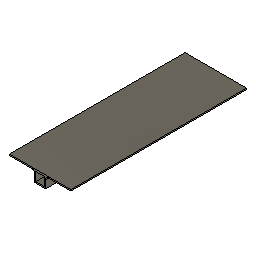
electronic_component_holder better (Autodesk Fusion 360 design; units mm, degrees)
Autodesk Fusion 360 part; units mm, degrees
sketch "Sketch1" plane through (0, 0, 0) normal (0, 0, 1) x (1, 0, 0)
  line L0 (0, 0) -> (17, 0)
  line L1 (17, 0) -> (17, 200)
  line L2 (17, 200) -> (0, 200)
  line L3 (0, 200) -> (0, 0)
  line L4 (5, 0) -> (5, 200)
  line L5 (12, 0) -> (12, 200)
  dimension "d1" = 17
  dimension "d2" = 200
  dimension "d3" = 200
  dimension "d4" = 7
  dimension "d5" = 200
  constraint horizontal L0
  constraint vertical L1
  constraint horizontal L2
  constraint vertical L3
  constraint coincident L0.start L3.end
  constraint coincident L0 L4.start
  constraint perpendicular L0 L5
  measures "d1" distance of L0.start L0.end
  measures "d2" distance of L0.start L2.end
  measures "d3" distance of L4.start L4.end
  measures "d4" distance of L4.start L5.start
  measures "d5" distance of L5.start L5.end
extrude "Extrude1" add sketch "Sketch1" along normal blind 5
sketch "Sketch2" plane through (0, 0, 5) normal (0, 0, 1) x (-1, 0, 0)
  line L0 (0, -200) -> (0, 0)
  line L1 (0, 0) -> (-17, 0)
  line L2 (-17, 0) -> (-17, -200)
  line L3 (-17, -200) -> (0, -200)
  line L4 (-5, 0) -> (-5, -200)
  line L5 (-12, 0) -> (-12, -200)
  dimension "d8" = 5
  dimension "d9" = 7
  dimension "d10" = 200
  dimension "d11" = 200
  constraint perpendicular L1 L4
  constraint perpendicular L1 L5
  measures "d8" distance of L0.end L4.start
  measures "d9" distance of L4.start L5.start
  measures "d10" distance of L4.start L4.end
  measures "d11" distance of L5.start L5.end
extrude "Extrude2" add sketch "Sketch2" along normal blind 12 contours L0 L1 L3 L4 | L1 L2 L3 L5
sketch "Sketch3" plane through (12, 0, 0) normal (-1, 0, 0) x (0, -1, 0)
  line L0 (-200, 5) -> (0, 5)
  line L1 (0, 5) -> (0, 17)
  line L2 (0, 17) -> (-200, 17)
  line L3 (-200, 17) -> (-200, 5)
  line L4 (0, 17) -> (0, 12)
  line L5 (0, 12) -> (-200, 12)
  dimension "d14" = 200
  constraint coincident L1.end L2.start
  constraint coincident L1 L4.end
  constraint perpendicular L2 L4
  constraint perpendicular L4 L5
  measures "d14" distance of L4.end L5.end
extrude "Extrude3" add sketch "Sketch3" along normal blind 7 contours L1 L2 L3 L4 L5
move_face "OffsetFaces1" offset -0.5 4 faces at (12, 133.3333, 9.6667) (9.6667, 66.6667, 12) (5, 133.3333, 9.6667) (7.3333, 133.3333, 5)
sketch "Sketch4" plane through (0, 0, 17) normal (0, 0, 1) x (-1, 0, 0)
  line L0 (-17, -200) -> (0, -200)
  line L1 (0, -200) -> (0, 0)
  line L2 (0, 0) -> (-17, 0)
  line L3 (-17, 0) -> (-17, -200)
  line L4 (25, 0) -> (25, -200)
  line L5 (-42, 0) -> (-42, -200)
  line L6 (25, -200) -> (-42, -200)
  line L7 (25, 0) -> (-42, 0)
  dimension "d18" = 25
  dimension "d19" = 25
  constraint perpendicular L5 L6
  constraint perpendicular L5 L7
  measures "d18" distance of L2.end L5.start
  measures "d19" distance of L1.end L4.start
extrude "Extrude4" add sketch "Sketch4" along normal blind 2.5
move_face "OffsetFaces2" offset -3 3 faces at (17, 133.3333, 11.3333) (5.6667, 133.3333, 0) (0, 133.3333, 5.6667)
move_face "MoveFace1" by (0, 0, 3) 4 faces at (7.1667, 133.3333, 12.5) (4.5, 133.3333, 9.8333) (7.1667, 133.3333, 4.5) (12.5, 133.3333, 9.8333)
extrude "Extrude5" cut 1 faces at (6.6667, 133.3333, 3) along direction (0, 0, 1) blind 3
extrude "Extrude6" cut 1 faces at (19.6667, 133.3333, 19.5) along direction (0, 0, -1) blind 1
move_face "OffsetFaces3" offset 0.5 4 faces at (12.5, 133.3333, 12.8333) (7.1667, 133.3333, 7.5) (7.1667, 133.3333, 15.5) (4.5, 133.3333, 12.8333)
move_face "OffsetFaces4" offset 1 4 faces at (5, 133.3333, 12.6667) (7.3333, 133.3333, 8) (12, 133.3333, 12.6667) (7.3333, 66.6667, 15)
move_face "OffsetFaces5" offset -0.5 4 faces at (11, 133.3333, 12.3333) (7.6667, 133.3333, 14) (6, 133.3333, 12.3333) (7.6667, 133.3333, 9)
move_face "OffsetFaces6" offset -0.5 3 faces at (14, 133.3333, 13.3333) (6.6667, 133.3333, 6) (3, 133.3333, 9.6667)
move_face "OffsetFaces7" offset -0.5 3 faces at (13.5, 133.3333, 13.5) (6.8333, 133.3333, 6.5) (3.5, 133.3333, 10)
move_face "OffsetFaces8" offset -0.5 3 faces at (13, 133.3333, 13.6667) (7, 133.3333, 7) (4, 133.3333, 10.3333)
move_face "MoveFace2" by (0, 0, 3) 4 faces at (11.5, 133.3333, 12.5) (7.5, 66.6667, 14.5) (7.5, 133.3333, 8.5) (5.5, 133.3333, 12.5)
move_face "OffsetFaces9" offset -3 1 faces at (7.1667, 133.3333, 7.5)
move_face "OffsetFaces10" offset -0.5 2 faces at (32.1667, 133.3333, 17) (-5.3333, 66.6667, 17)
extrude "Extrude7" add 1 faces at (7.1667, 133.3333, 10.5) along direction (0, 0, -1) blind 0.5
move_face "MoveFace3" by (0, 0, -0.5) 4 faces at (11.5, 133.3333, 15.5) (7.5, 66.6667, 17.5) (5.5, 133.3333, 15.5) (7.5, 133.3333, 11.5)
move_face "OffsetFaces11" offset -4.5 1 faces at (42, 133.3333, 18.1667)
move_face "OffsetFaces12" offset -4.5 1 faces at (-25, 133.3333, 18.1667)
move_face "OffsetFaces13" offset 50 1 faces at (7.1667, 0, 18.1667)
move_face "OffsetFaces14" offset -0.5 4 faces at (11.5, 116.6667, 15) (7.5, 116.6667, 11) (5.5, 116.6667, 15) (7.5, 116.6667, 17)
move_face "OffsetFaces15" offset 0.5 3 faces at (12.5, 116.6667, 15) (7.1667, 116.6667, 10) (4.5, 116.6667, 12.5)
move_face "OffsetFaces16" offset 0.5 1 faces at (7, 116.6667, 9.5)
move_face "MoveFace4" by (0, 0, -0.5) 4 faces at (12, 116.6667, 15.1667) (7.3333, 116.6667, 10.5) (5, 116.6667, 15.1667) (7.3333, 116.6667, 17.5)
move_face "OffsetFaces17" offset 0.5 4 faces at (12, 116.6667, 14.6667) (7.3333, 116.6667, 17) (5, 116.6667, 14.6667) (7.3333, 116.6667, 10)
move_face "MoveFace5" by (0, 0, 0.5) 4 faces at (5.5, 116.6667, 14.5) (7.5, 116.6667, 10.5) (11.5, 116.6667, 14.5) (7.5, 116.6667, 16.5)
move_face "OffsetFaces18" offset -0.5 1 faces at (7, 116.6667, 9)
move_face "OffsetFaces19" offset -0.02 1 faces at (7.5, 116.6667, 11)
move_face "OffsetFaces20" offset -0.2 2 faces at (11.5, 116.6667, 14.9933) (5.5, 116.6667, 14.9933)
move_face "OffsetFaces21" offset -0.18 2 faces at (7.4333, 116.6667, 17) (7.4333, 116.6667, 10.98)
move_face "OffsetFaces22" offset 0.18 1 faces at (7.4333, 116.6667, 17.18)
move_face "OffsetFaces23" offset 0.1 2 faces at (11.7, 116.6667, 14.9333) (5.3, 116.6667, 14.9333)
move_face "OffsetFaces24" offset 0.1 2 faces at (13, 116.6667, 14.8333) (4, 116.6667, 12.1667)
move_face "OffsetFaces25" offset 0.2 1 faces at (6.9667, 116.6667, 9.5)
move_face "OffsetFaces26" offset -1 1 faces at (18.1667, 116.6667, 18.5)
move_face "OffsetFaces27" offset -202.2 1 faces at (9.5333, -50, 9.8)
move_face "OffsetFaces28" offset 1 1 faces at (9.5333, 152.2, 9.8)
move_face "OffsetFaces29" offset -0.4 4 faces at (11.6, 183.7333, 14.9333) (9.5333, 183.7333, 17) (5.4, 183.7333, 14.9333) (7.4667, 183.7333, 10.8)
extrude "Extrude8" cut 1 faces at (6.9667, 183.7333, 9.3) along direction (0, 0, 1) blind 0.1
extrude "Extrude9" cut 1 faces at (13.1, 183.7333, 14.8) along direction (-1, 0, 0) blind 0.1
extrude "Extrude10" cut 1 faces at (3.9, 167.4667, 14.8) along direction (1, 0, 0) blind 0.1
extrude "Extrude11" add 1 faces at (10, 183.7333, 17.5) along direction (0, 0, 1) blind 0.9
sketch "Sketch5" plane through (13, 0, 0) normal (1, 0, 0) x (0, 1, 0)
  line L0 (151.2, 9.4) -> (200, 9.4)
  line L1 (200, 9.4) -> (200, 18.4)
  line L2 (200, 18.4) -> (151.2, 18.4)
  line L3 (151.2, 18.4) -> (151.2, 9.4)
  line L4 (151.2, 18.4) -> (151.2, 17.4)
  line L5 (151.2, 17.4) -> (200, 17.4)
  dimension "d64" = 1
  constraint coincident L2.end L3.start
  constraint perpendicular L2 L4
  constraint coincident L1 L5.end
  constraint perpendicular L1 L5
  measures "d64" distance of L2.end L4.end
extrude "Extrude12" add sketch "Sketch5" along normal blind 5 contours L1 L2 L3 L4 L5
sketch "Sketch6" plane through (4, 0, 0) normal (-1, 0, 0) x (0, -1, 0)
  line L0 (-200, 9.4) -> (-151.2, 9.4)
  line L1 (-151.2, 9.4) -> (-151.2, 18.4)
  line L2 (-151.2, 18.4) -> (-200, 18.4)
  line L3 (-200, 18.4) -> (-200, 9.4)
  line L4 (-151.2, 18.4) -> (-151.2, 17.4)
  line L5 (-151.2, 17.4) -> (-200, 17.4)
  dimension "d67" = 1
  constraint coincident L1.end L2.start
  constraint perpendicular L2 L4
  constraint coincident L3 L5.end
  constraint perpendicular L3 L5
  measures "d67" distance of L1.end L4.end
extrude "Extrude13" add sketch "Sketch6" along normal blind 5 contours L1 L2 L3 L4 L5
fillet "Fillet1" radius 2 1 edges at (4, 175.6, 17.4)
fillet "Fillet2" radius 2 1 edges at (13, 175.6, 17.4)
extrude "Extrude14" add 1 faces at (18, 183.7333, 17.7333) along direction (1, 0, 0) blind 5
extrude "Extrude15" add 1 faces at (-1, 167.4667, 17.7333) along direction (-1, 0, 0) blind 5
extrude "Extrude16" cut 1 faces at (13.3333, 183.7333, 18.4) along direction (0, 0, -1) blind 0.5
extrude "Extrude17" add 1 faces at (7.3333, 183.7333, 17.4) along direction (0, 0, -1) blind 0.5
extrude "Extrude18" cut 1 faces at (7.3333, 183.7333, 10.4) along direction (0, 0, -1) blind 0.5
extrude "Extrude19" add 1 faces at (7, 167.4667, 9.4) along direction (0, 0, -1) blind 0.5
extrude "Extrude20" add 1 faces at (23, 183.7333, 17.5667) along direction (1, 0, 0) blind 10
extrude "Extrude21" add 1 faces at (-6, 167.4667, 17.5667) along direction (-1, 0, 0) blind 10
extrude "Extrude22" add 1 faces at (16.6667, 183.7333, 17.9) along direction (0, 0, 1) blind 1.5
extrude "Extrude23" cut 1 faces at (16.6667, 183.7333, 19.4) along direction (0, 0, -1) blind 1
extrude "Extrude24" add 1 faces at (6.3333, 200, 18.0667) along direction (0, 1, 0) blind 125.2
extrude "Extrude25" cut 1 faces at (6.3333, 325.2, 18.0667) along direction (0, -1, 0) blind 34
equation "d94 = 140 mm - 14.8 mm"
